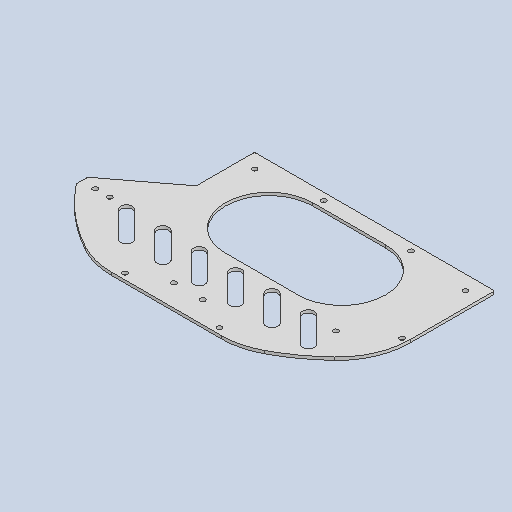
# Autodesk Inventor part: T2.0_frame-base3
Saved by Autodesk Inventor 2025.1 (Build 291241020, 241B)
## iProperties
Created: 2024-06-26
Part Number: T2.0_frame-base3
Material: 一般
Document SubType Name: Sheet Metal
Designer: 8326d
Density: 1 g/cm^3
Sheet Metal Rule: Default_mm
Appearance: 既定
Author: 8326d
Autodesk Inventor part; units mm, degrees
ref_plane "YZ Plane" through (0, 0, 0) normal (1, 0, 0) x (0, 1, 0)
ref_plane "XZ Plane" through (0, 0, 0) normal (0, 1, 0) x (-1, 0, 0)
ref_plane "XY Plane" through (0, 0, 0) normal (0, 0, 1) x (1, 0, 0)
sketch "スケッチ1" plane through (0, 0, 0) normal (0, 1, 0) x (-1, 0, 0)
  circle A0 centre (0, 0) radius 130
  dimension "d0" = 260
  measures "d0" diameter of A0
extrude "プレート1" add sketch "スケッチ1" along normal blind 2
sketch "スケッチ4" plane through (0, 2, 0) normal (0, 1, 0) x (1, 0, 0)
  circle A0 centre (0, 0) radius 130 projected
  line L0 (-106.1838, 75) -> (-60, 40)
  line L1 (-60, 40) -> (-60, -40)
  line L2 (-60, -40) -> (-106.1838, -75)
  point P0 (-60, 0)
  dimension "d17" = 40
  dimension "d18" = 75
  dimension "d19" = 60
  constraints: 6 end point, 2 point on circle, 1 horizontal alignment, 1 midpoint, 1 vertical, 1 vertical alignment
  measures "d17" vertical distance of L1.end point (0, 0)
  measures "d18" vertical distance of point (0, 0) L0.start
  measures "d19" distance from line of point (0, 0) L1
extrude "押し出し2" cut sketch "スケッチ4" against normal through all contours L0 L1 L2 A0 picked at (-83.3333, 0)
sketch "スケッチ7" plane through (0, 2, 0) normal (0, 1, 0) x (1, 0, 0)
  arc A0 (-106.1838, -75) -> (-106.1838, 75) centre (0, 0) ccw projected
  line L0 (-48.7827, 120.5) -> (48.7827, 120.5)
  line L1 (-48.7827, -120.5) -> (48.7827, -120.5)
  line L2 (105, -76.6485) -> (105, 76.6485)
  dimension "d68" = 120.5
  dimension "d69" = 120.5
  dimension "d70" = 105
  constraints: 6 end point, 6 point on circle, 1 horizontal, 1 parallel, 1 perpendicular
  measures "d68" distance from line of point (0, 0) L0
  measures "d69" distance from line of L1 point (0, 0)
  measures "d70" distance from line of point (0, 0) L2
extrude "押し出し4" cut sketch "スケッチ7" against normal through all
fillet "フィレット4" radius 50 6 edges at (-48.7827, 1, 120.5) (48.7827, 1, 120.5) (105, 1, -76.6485) (105, 1, 76.6485) (-48.7827, 1, -120.5) (48.7827, 1, -120.5)
sketch "スケッチ9" plane through (0, 2, 0) normal (0, 1, 0) x (1, 0, 0)
  line L0 (101.5, -60) -> (101.5, 60) construction
  line L1 (101.5, -60) -> (221.5, -60) construction
  line L2 (105, -58.0948) -> (105, 58.0948) construction
  point P0 (0, 0)
  point P1 (101.5, 0)
  dimension "d71" = 120
  dimension "d72" = 90
  dimension "d73" = 3.5
  constraints: 4 end point, 1 horizontal, 1 horizontal alignment, 1 midpoint, 1 perpendicular, 1 vertical
  measures "d71" distance of L0.start L0.end
  measures "d72" angle of L1 L0
  measures "d73" distance between parallel lines of L2 L0
hole "穴4" at (101.5, 2, 60) at (101.5, 2, -60) direction (0, -1, 0) diameter 3.5 depth 2 tip angle 118
sketch "スケッチ10" plane through (0, 2, 0) normal (0, 1, 0) x (1, 0, 0)
  line L0 (10, -105.5) -> (-10, -105.5) construction
  line L1 (-10, -105.5) -> (-10, 105.5) construction
  line L2 (-10, 105.5) -> (10, 105.5) construction
  line L3 (10, 105.5) -> (10, -105.5) construction
  line L4 (10, -105.5) -> (-10, 105.5) construction
  line L5 (-10, -105.5) -> (10, 105.5) construction
  point P0 (0, 0)
  dimension "d81" = 20
  dimension "d82" = 211
  constraints: 12 end point, 2 midpoint, 2 parallel, 1 horizontal, 1 perpendicular
  measures "d81" distance of L1.end L2.end
  measures "d82" distance of L0.end L1.end
hole "穴5" at (-10, 2, 105.5) at (10, 2, 105.5) at (10, 2, -105.5) at (-10, 2, -105.5) direction (0, -1, 0) diameter 3.5 depth 2 tip angle 118
sketch "スケッチ11" plane through (0, 2, 0) normal (0, 1, 0) x (1, 0, 0)
  line L0 (-32.5, 116.5) -> (32.5, 116.5) construction
  line L1 (-32.5, 116.5) -> (32.5, 116.5) construction
  line L2 (37.812, 120.5) -> (-37.812, 120.5) construction
  point P0 (0, 0)
  point P1 (0, 116.5)
  dimension "d90" = 65
  dimension "d91" = 0
  dimension "d92" = 4
  constraints: 4 end point, 2 horizontal, 1 collinear, 1 midpoint, 1 vertical alignment
  measures "d90" distance of L0.start L0.end
  measures "d91" distance between parallel lines of L0 L1
  measures "d92" distance between parallel lines of L2 L0
hole "穴6" at (32.5, 2, -116.5) at (-32.5, 2, -116.5) direction (0, -1, 0) diameter 3.5 end through all
mirror "ミラー3" about plane through (0, 0, 0) normal (0, 0, 1) of "穴6"
sketch "スケッチ12" plane through (0, 2, 0) normal (0, 1, 0) x (1, 0, 0)
  line L0 (-50, 10) -> (-50, -10) construction
  line L1 (-50, 10) -> (-30, 10) construction
  line L2 (-60, 40) -> (-60, -40) construction
  point P0 (0, 0)
  point P1 (-50, 0)
  dimension "d100" = 20
  dimension "d101" = 90
  dimension "d102" = 10
  constraints: 4 end point, 1 horizontal, 1 horizontal alignment, 1 midpoint, 1 perpendicular, 1 vertical
  measures "d100" distance of L0.start L0.end
  measures "d101" angle of L0 L1
  measures "d102" distance between parallel lines of L2 L0
hole "穴7" at (-50, 2, 10) at (-50, 2, -10) direction (0, -1, 0) diameter 3.5 end through all
sketch "スケッチ13" plane through (0, 2, 0) normal (0, 1, 0) x (1, 0, 0)
  line L0 (-10, 40) -> (40, 40) construction
  line L1 (-10, 10) -> (40, 10)
  line L2 (40, 70) -> (-10, 70)
  arc A0 (-10, 70) -> (-10, 10) centre (-10, 40) ccw
  arc A1 (40, 10) -> (40, 70) centre (40, 40) ccw
  point P0 (0, 0)
  point P1 (15, 40)
  dimension "d110" = 40
  dimension "d111" = 60
  dimension "d112" = 50
  dimension "d113" = 15
  constraints: 8 end point, 4 point on circle, 4 tangent, 2 centre point, 1 horizontal, 1 midpoint, 1 parallel
  measures "d110" distance from line of point (0, 0) L0
  measures "d111" distance between parallel lines of L2 L1
  measures "d112" distance of L0.start L0.end
  measures "d113" horizontal distance of point (0, 0) point (15, 40)
extrude "押し出し5" cut sketch "スケッチ13" against normal through all
sketch "スケッチ14" plane through (0, 2, 0) normal (0, 1, 0) x (1, 0, 0)
  line L0 (72.6777, 95.6777) -> (55, 78) construction
  line L1 (75.5061, 92.8492) -> (57.8284, 75.1716)
  line L2 (52.1716, 80.8284) -> (69.8492, 98.5061)
  arc A0 (75.5061, 92.8492) -> (69.8492, 98.5061) centre (72.6777, 95.6777) ccw
  arc A1 (52.1716, 80.8284) -> (57.8284, 75.1716) centre (55, 78) ccw
  line L3 (-10, 70) -> (40, 70) projected
  point P0 (0, 0)
  point P1 (63.8388, 86.8388)
  dimension "d116" = 135
  dimension "d117" = 8
  dimension "d118" = 25
  dimension "d119" = 4
  dimension "d120" = 15
  constraints: 8 end point, 4 point on circle, 4 tangent, 2 centre point, 1 midpoint, 1 parallel
  measures "d116" angle of L3 L0
  measures "d117" distance from line of L3 L0.end
  measures "d118" distance of L0.start L0.end
  measures "d119" radius of A0
  measures "d120" horizontal distance of L3.end L0.end
extrude "押し出し6" cut sketch "スケッチ14" against normal through all
pattern_linear "矩形状パターン1" count 6 spacing 25 along (-1, 0, 0) of "押し出し6"
mirror "ミラー4" about plane through (0, 0, 0) normal (0, 0, 1) of "押し出し5", "押し出し6", "矩形状パターン1"
sketch "スケッチ15" plane through (0, 0, 0) normal (0, -1, 0) x (1, 0, 0)
  arc A0 (73.6766, 79.5874) -> (73.6766, 77.4126) centre (74.2931, 78.5) ccw projected
  arc A1 (74.9095, -79.5874) -> (74.9095, -77.4126) centre (74.2931, -78.5) ccw projected
  point P0 (0, 0)
hole "穴8" at (74.2931, 0, -78.5) at (74.2931, 0, 78.5) direction (0, 1, 0) diameter 3.5 end through all
sketch "スケッチ16" plane through (0, 2, 0) normal (0, 1, 0) x (1, 0, 0)
  arc A0 (-61.4446, 114.5625) -> (-106.1838, 75) centre (0, 0) ccw projected
  arc A1 (-106.1838, -75) -> (-61.4446, -114.5625) centre (0, 0) ccw projected
  line L0 (-102.4695, 80) -> (-102.4695, -80)
  line L1 (-102.4695, 80) -> (57.5305, 80) construction
  line L2 (-106.1838, 75) -> (-60, 40) projected
  line L3 (-60, -40) -> (-106.1838, -75) projected
  point P0 (-102.4695, 72.1852)
  point P1 (-102.4695, -72.1852)
  dimension "d133" = 160
  dimension "d134" = 90
  constraints: 4 end point, 2 point on circle, 1 horizontal, 1 perpendicular, 1 vertical
  measures "d133" distance of L0.start L0.end
  measures "d134" angle of L0 L1
extrude "押し出し7" cut sketch "スケッチ16" against normal through all
sketch "スケッチ17" plane through (0, 2, 0) normal (0, 1, 0) x (1, 0, 0)
  line L0 (-92.9695, 76.5) -> (-82.9695, 76.5) construction
  line L1 (-82.9695, 76.5) -> (-82.9695, -76.5) construction
  line L2 (-82.9695, -76.5) -> (-92.9695, -76.5) construction
  line L3 (-92.9695, -76.5) -> (-92.9695, 76.5) construction
  line L4 (-92.9695, 76.5) -> (-82.9695, -76.5) construction
  line L5 (-82.9695, 76.5) -> (-92.9695, -76.5) construction
  line L6 (-102.4695, 80) -> (-102.4695, 72.1852) construction
  point P0 (0, 0)
  point P1 (-87.9695, 0)
  dimension "d137" = 10
  dimension "d138" = 153
  dimension "d139" = 9.5
  constraints: 12 end point, 4 coincident, 2 midpoint, 2 parallel, 1 horizontal, 1 horizontal alignment, 1 perpendicular
  measures "d137" distance of L1.end L2.end
  measures "d138" distance of L0.end L1.end
  measures "d139" distance between parallel lines of L6 L3
hole "穴9" at (-92.9695, 2, -76.5) at (-82.9695, 2, -76.5) at (-92.9695, 2, 76.5) at (-82.9695, 2, 76.5) direction (0, -1, 0) diameter 3.5 end through all
fillet "フィレット5" radius 2 6 edges at (-102.4695, 1, -72.1852) (-102.4695, 1, 80) (-102.4695, 1, -80) (-60, 1, -40) (-60, 1, 40) (-102.4695, 1, 72.1852)
sketch "スケッチ18" plane through (0, 2, 0) normal (0, 1, 0) x (1, 0, 0)
  line L0 (105, -58.0948) -> (105, 58.0948) projected
  line L1 (-60, 39.0062) -> (-60, -39.0062) projected
  line L2 (-60, 0) -> (105, 0) construction
  circle A0 centre (-50, 10) radius 1.75 construction
  line L3 (95, -10) -> (-50, -10) construction
  line L4 (-50, -10) -> (-50, 10) construction
  line L5 (-50, 10) -> (95, 10) construction
  line L6 (95, 10) -> (95, -10) construction
  line L7 (95, -10) -> (-50, 10) construction
  line L8 (-50, -10) -> (95, 10) construction
  line L9 (52.5, -5) -> (-7.5, -5) construction
  line L10 (-7.5, -5) -> (-7.5, 5) construction
  line L11 (-7.5, 5) -> (52.5, 5) construction
  line L12 (52.5, 5) -> (52.5, -5) construction
  line L13 (52.5, -5) -> (-7.5, 5) construction
  line L14 (-7.5, -5) -> (52.5, 5) construction
  point P0 (0, 0)
  point P1 (22.5, 0)
  point P2 (22.5, 0)
  dimension "d148" = 60
  dimension "d149" = 10
  constraints: 26 end point, 8 midpoint, 4 parallel, 2 horizontal, 2 perpendicular
  measures "d148" distance of L10.end L11.end
  measures "d149" distance of L9.end L10.end
hole "穴10" at (95, 2, 10) at (95, 2, -10) at (52.5, 2, 5) at (52.5, 2, -5) at (-7.5, 2, -5) at (-7.5, 2, 5) direction (0, -1, 0) diameter 3.5 end through all
sketch "スケッチ19" plane through (0, 2, 0) normal (0, 1, 0) x (1, 0, 0)
  line L0 (-60, 39.0062) -> (-60, -39.0062) projected
  arc A0 (-60, 39.0062) -> (-60.792, 40.6002) centre (-62, 39.0062) ccw projected
  line L1 (-101.6775, 71.5849) -> (-60.792, 40.6002) projected
  arc A1 (-102.4695, 73.1789) -> (-101.6775, 71.5849) centre (-100.4695, 73.1789) ccw projected
  line L2 (-102.4695, 79.3088) -> (-102.4695, 73.1789) projected
  arc A2 (-102.0393, 80.548) -> (-102.4695, 79.3088) centre (-100.4695, 79.3088) ccw projected
  arc A3 (-61.4446, 114.5625) -> (-102.0393, 80.548) centre (0, 0) ccw projected
  arc A4 (-37.812, 120.5) -> (-61.4446, 114.5625) centre (-37.812, 70.5) ccw projected
  line L3 (37.812, 120.5) -> (-37.812, 120.5) projected
  arc A5 (61.4446, 114.5625) -> (37.812, 120.5) centre (37.812, 70.5) ccw projected
  arc A6 (89.375, 94.404) -> (61.4446, 114.5625) centre (0, 0) ccw projected
  arc A7 (105, 58.0948) -> (89.375, 94.404) centre (55, 58.0948) ccw projected
  line L4 (105, -58.0948) -> (105, 58.0948) projected
  line L5 (-60, 0) -> (105, 0)
  constraints: 2 end point, 2 midpoint
extrude "押し出し8" cut sketch "スケッチ19" against normal through all
fillet "フィレット6" radius 1 2 edges at (-60, 1, 0) (105, 1, 0)
sketch "スケッチ20" plane through (0, 0, 0) normal (0, 1, 0) x (-1, 0, 0)
  line L0 (115.5948, 100.5744) -> (-72.3437, 168.9784)
  line L1 (-72.3437, 168.9784) -> (-130.4866, 9.2322)
  line L2 (-130.4866, 9.2322) -> (57.4519, -59.1718)
  line L3 (57.4519, -59.1718) -> (115.5948, 100.5744)
  line L4 (-104, 0) -> (59, 0) projected
  point P0 (0, 0)
  dimension "d161" = 200
  dimension "d162" = 20
  constraints: 8 end point, 2 parallel, 1 perpendicular
  measures "d161" distance of L0.start L0.end
  measures "d162" angle of L4 L2
equation "\"d69\" = d68"
equation "\"d79\" = Thickness"
equation "\"d88\" = Thickness"
equation "\"d98\" = Thickness"
equation "\"d108\" = Thickness"
equation "\"d131\" = Thickness"
equation "\"d145\" = Thickness"
equation "\"d155\" = Thickness"
equation "\"d1\" = Thickness"
equation "\"BendRadius\" = Thickness"
equation "\"BendReliefWidth\" = Thickness"
equation "\"BendReliefDepth\" = 0.5 * Thickness"
equation "\"CornerReliefSize\" = 4 * Thickness"
equation "\"MinimumRemnant\" = 2 * Thickness"
equation "\"TransitionRadius\" = BendRadius"
equation "\"JacobiRadiusSize\" = BendRadius"
equation "\"GapSize\" = Thickness"
equation "\"Thickness\" = 2"
